Autodesk Inventor part; units mm, degrees
(part 2 of 2)
sketch "Sketch21" plane through (0, 0, 3) normal (0, 0, 1) x (1, 0, 0)
  line L0 (-66, -139.4) -> (-40.5, -139.4) projected
  arc A0 (-71.75, -135.4) -> (-68.25, -135.4) centre (-70, -135.4) ccw projected
  arc A1 (-68.25, -132.4) -> (-71.75, -132.4) centre (-70, -132.4) ccw projected
  line L1 (-71.75, -135.4) -> (-71.75, -132.4) projected
  line L2 (-68.25, -132.4) -> (-68.25, -135.4) projected
  arc A2 (-66, -139.4) -> (-69, -142.4) centre (-66, -142.4) ccw projected
  line L3 (-69, -186.9) -> (-69, -142.4) projected
  line L4 (-45.75, -135.2) -> (-45.75, -132.2) projected
  arc A3 (-42.25, -132.2) -> (-45.75, -132.2) centre (-44, -132.2) ccw projected
  line L5 (-42.25, -132.2) -> (-42.25, -135.2) projected
  arc A4 (-45.75, -135.2) -> (-42.25, -135.2) centre (-44, -135.2) ccw projected
  arc A5 (-34.5, -132.6) -> (-37.5, -135.6) centre (-34.5, -135.6) ccw projected
  arc A6 (-40.5, -139.4) -> (-37.5, -136.4) centre (-40.5, -136.4) ccw projected
  line L6 (-37.5, -136.4) -> (-37.5, -135.6) projected
  line L7 (-34.5, -132.6) -> (58.5, -132.6) projected
  arc A7 (61.5, -135.6) -> (58.5, -132.6) centre (58.5, -135.6) ccw projected
  line L8 (66.25, -135.4) -> (66.25, -132.4) projected
  arc A8 (69.75, -132.4) -> (66.25, -132.4) centre (68, -132.4) ccw projected
  line L9 (69.75, -132.4) -> (69.75, -135.4) projected
  arc A9 (66.25, -135.4) -> (69.75, -135.4) centre (68, -135.4) ccw projected
  arc A10 (71.75, -142.2) -> (68.25, -142.2) centre (70, -142.2) ccw projected
  line L10 (68.25, -145.2) -> (68.25, -142.2) projected
  line L11 (71.75, -142.2) -> (71.75, -145.2) projected
  arc A11 (68.25, -145.2) -> (71.75, -145.2) centre (70, -145.2) ccw projected
  line L12 (61.5, -135.6) -> (61.5, -148.7) projected
  arc A12 (61.5, -148.7) -> (64.5, -151.7) centre (64.5, -148.7) ccw projected
  line L13 (64.5, -151.7) -> (66, -151.7) projected
  arc A13 (69, -154.7) -> (66, -151.7) centre (66, -154.7) ccw projected
  line L14 (69, -154.7) -> (69, -199.4) projected
  arc A14 (66, -202.4) -> (69, -199.4) centre (66, -199.4) ccw projected
  line L15 (66, -202.4) -> (39.9991, -202.4) projected
  arc A15 (71.75, -206.2) -> (68.25, -206.2) centre (70, -206.2) ccw projected
  line L16 (68.25, -209.2) -> (68.25, -206.2) projected
  line L17 (71.75, -206.2) -> (71.75, -209.2) projected
  arc A16 (68.25, -209.2) -> (71.75, -209.2) centre (70, -209.2) ccw projected
  arc A17 (39.9991, -202.4) -> (37.2495, -204.2) centre (39.9991, -205.4) ccw projected
  arc A18 (34.5, -206) -> (37.2495, -204.2) centre (34.5, -203) ccw projected
  line L18 (34.5, -206) -> (-58.5, -206) projected
  line L19 (42.25, -209.4) -> (42.25, -206.4) projected
  arc A19 (45.75, -206.4) -> (42.25, -206.4) centre (44, -206.4) ccw projected
  line L20 (45.75, -206.4) -> (45.75, -209.4) projected
  arc A20 (42.25, -209.4) -> (45.75, -209.4) centre (44, -209.4) ccw projected
  arc A21 (-61.5, -203) -> (-58.5, -206) centre (-58.5, -203) ccw projected
  line L21 (-61.5, -203) -> (-61.5, -192.9) projected
  arc A22 (-61.5, -192.9) -> (-64.5, -189.9) centre (-64.5, -192.9) ccw projected
  arc A23 (-69, -186.9) -> (-66, -189.9) centre (-66, -186.9) ccw projected
  line L22 (-64.5, -189.9) -> (-66, -189.9) projected
  arc A24 (-68, -196.4) -> (-72, -196.4) centre (-70, -196.4) ccw projected
  line L23 (-68, -196.4) -> (-68, -199.4) projected
  line L24 (-72, -199.4) -> (-72, -196.4) projected
  arc A25 (-72, -199.4) -> (-68, -199.4) centre (-70, -199.4) ccw projected
  arc A26 (-66.25, -206.2) -> (-69.75, -206.2) centre (-68, -206.2) ccw projected
  line L25 (-69.75, -209.2) -> (-69.75, -206.2) projected
  line L26 (-66.25, -206.2) -> (-66.25, -209.2) projected
  arc A27 (-69.75, -209.2) -> (-66.25, -209.2) centre (-68, -209.2) ccw projected
  point P0 (0, 0)
equation "\"d7\" = d6"
equation "\"d8\" = d6"
equation "\"d9\" = d6"
equation "\"d12\" = d11"
equation "\"d32\" = d29"
equation "\"d48\" = d49"
equation "\"d52\" = d51"
equation "\"d53\" = d51"
equation "\"d54\" = d49"
equation "\"d56\" = d51"
equation "\"d57\" = d49"
equation "\"d58\" = d51"
equation "\"d59\" = d51"
equation "\"d84\" = d70 + d69"
